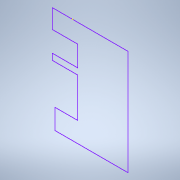
# Autodesk Inventor part: PlacaBase
Saved by Autodesk Inventor 2021 (Build 250183000, 183)
## iProperties
Created: 2022-10-28
Part Number: PlacaBase
Material: Generic
Document SubType Name: Modeling
Designer: zulet
Density: 1 g/cm^3
Appearance: Default
Author: zulet
Autodesk Inventor part; units mm, degrees
ref_plane "YZ Plane" through (0, 0, 0) normal (1, 0, 0) x (0, 1, 0)
ref_plane "XZ Plane" through (0, 0, 0) normal (0, 1, 0) x (-1, 0, 0)
ref_plane "XY Plane" through (0, 0, 0) normal (0, 0, 1) x (1, 0, 0)
sketch "Sketch1" plane through (0, 0, 0) normal (0, 0, 1) x (1, 0, 0)
  line L0 (-24.2798, -142.4572) -> (74.9078, -142.4572)
  line L1 (74.9078, -142.4572) -> (74.9078, 0)
  line L2 (74.9078, 0) -> (-27.6862, 0)
  line L3 (-27.6862, 0) -> (-27.6862, -25.6363)
  line L4 (-27.6862, -25.6363) -> (6.779, -25.6363)
  line L5 (6.779, -25.6363) -> (6.779, -53.489)
  line L6 (6.779, -53.489) -> (-27.6862, -53.489)
  line L7 (-27.6862, -53.489) -> (-27.6862, -61.9049)
  line L8 (-27.6862, -61.9049) -> (6.779, -61.9049)
  line L9 (6.779, -61.9049) -> (6.779, -115.2057)
  line L10 (6.779, -115.2057) -> (-24.2798, -115.2057)
  line L11 (-24.2798, -115.2057) -> (-24.2798, -142.4572)
  point P0 (0, 0)
  constraints: 24 end point, 9 perpendicular, 4 point on line, 1 horizontal
extrude "Extrusion1" add sketch "Sketch1" along normal blind 5
body "Solid1"
